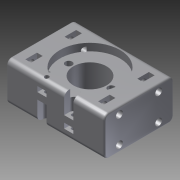
# Autodesk Inventor part: Z move middle
Saved by Autodesk Inventor 2012 (Build 160160000, 160)
## iProperties
Created: 2013-02-05
Part Number: Z move middle
Material: Default
Document SubType Name: Modeling
Designer: mce
Density: 1 g/cm^3
Mass: 44.0832 g
Surface Area: 145.334 cm^2
Volume: 44.0832 cm^3
Author: mce
Autodesk Inventor part; units mm, degrees
ref_plane "YZ Plane" through (0, 0, 0) normal (1, 0, 0) x (0, 1, 0)
ref_plane "XZ Plane" through (0, 0, 0) normal (0, 1, 0) x (-1, 0, 0)
ref_plane "XY Plane" through (0, 0, 0) normal (0, 0, 1) x (1, 0, 0)
sketch "Sketch1" plane through (0, 0, 0) normal (0, 0, 1) x (1, 0, 0)
  line L0 (0, 0) -> (60, 0)
  line L1 (60, 0) -> (60, 42.4)
  line L2 (60, 42.4) -> (0, 42.4)
  line L3 (0, 42.4) -> (0, 0)
  circle A0 centre (30, 21.2) radius 10.15
  dimension "d0" = 42.4
  dimension "d1" = 60
  dimension "d2" = 20.3
  dimension "d3" = 21.2
  dimension "d4" = 30
  constraints: 8 end point, 2 horizontal, 2 vertical, 1 centre point
  measures "d0" distance of L2.end L0.start
  measures "d1" distance of L0.start L0.end
  measures "d2" diameter of A0
  measures "d3" distance from line of L2 A0.centre
  measures "d4" distance from line of L3 A0.centre
extrude "Extrusion1" add sketch "Sketch1" along normal blind 24
sketch "Sketch2" plane through (0, 0, 0) normal (-1, 0, 0) x (0, 0, 1)
  line L0 (24, 0) -> (24, 42.4) projected
  line L1 (0, 42.4) -> (24, 42.4) projected
  line L2 (0, 42.4) -> (0, 0) projected
  line L3 (0, 0) -> (24, 0) projected
  circle A0 centre (4, 33.2) radius 2.1
  circle A1 centre (20, 33.2) radius 2.1
  circle A2 centre (20, 9.2) radius 2.1
  circle A3 centre (4, 9.2) radius 2.1
  dimension "d7" = 4.2
  dimension "d8" = 9.2
  dimension "d9" = 9.2
  dimension "d10" = 9.2
  dimension "d11" = 9.2
  dimension "d12" = 4
  dimension "d13" = 4
  dimension "d14" = 4
  dimension "d15" = 4
  constraints: 4 centre point, 3 equal radius
  measures "d7" diameter of A0
  measures "d8" distance from line of L1 A0.centre
  measures "d9" distance from line of L1 A1.centre
  measures "d10" distance from line of L3 A2.centre
  measures "d11" distance from line of L3 A3.centre
  measures "d12" distance from line of L2 A0.centre
  measures "d13" distance from line of L2 A3.centre
  measures "d14" distance from line of L0 A2.centre
  measures "d15" distance from line of L0 A1.centre
extrude "Extrusion2" cut sketch "Sketch2" against normal blind 16 contours A0 | A1 | A2 | A3
sketch "Sketch3" plane through (60, 0, 0) normal (1, 0, 0) x (0, 0, -1)
  line L0 (-24, 42.4) -> (-24, 0) projected
  line L1 (0, 0) -> (-24, 0) projected
  line L2 (0, 0) -> (0, 42.4) projected
  line L3 (0, 42.4) -> (-24, 42.4) projected
  circle A0 centre (-20, 33.2) radius 2.1
  circle A1 centre (-4, 33.2) radius 2.1
  circle A2 centre (-4, 9.2) radius 2.1
  circle A3 centre (-20, 9.2) radius 2.1
  dimension "d18" = 4.2
  dimension "d19" = 4
  dimension "d20" = 4
  dimension "d21" = 4
  dimension "d22" = 4
  dimension "d23" = 9.2
  dimension "d24" = 9.2
  dimension "d25" = 9.2
  dimension "d26" = 9.2
  constraints: 4 centre point, 3 equal radius
  measures "d18" diameter of A0
  measures "d19" distance from line of L0 A0.centre
  measures "d20" distance from line of L0 A3.centre
  measures "d21" distance from line of L2 A2.centre
  measures "d22" distance from line of L2 A1.centre
  measures "d23" distance from line of L3 A0.centre
  measures "d24" distance from line of L3 A1.centre
  measures "d25" distance from line of L1 A2.centre
  measures "d26" distance from line of L1 A3.centre
extrude "Extrusion3" cut sketch "Sketch3" against normal blind 16 contours A0 | A1 | A2 | A3
fillet "Fillet1" radius 3 4 edges at (30, 42.4, 0) (30, 0, 0) (30, 42.4, 24) (30, 0, 24)
fillet "Fillet2" radius 1 16 edges at (60, 21.2, 24) (60, 0.8787, 23.1213) (60, 0, 12) (60, 0.8787, 0.8787) (60, 21.2, 0) (60, 41.5213, 0.8787) (60, 42.4, 12) (60, 41.5213, 23.1213) (0, 41.5213, 23.1213) (0, 42.4, 12) (0, 41.5213, 0.8787) (0, 21.2, 0) (0, 0.8787, 0.8787) (0, 0, 12) (0, 0.8787, 23.1213) (0, 21.2, 24)
sketch "Sketch4" plane through (0, 0, 24) normal (0, 0, 1) x (1, 0, 0)
  line L0 (6, 36.75) -> (9.5, 36.75)
  line L1 (9.5, 36.75) -> (9.5, 29.65)
  line L2 (9.5, 29.65) -> (6, 29.65)
  line L3 (6, 29.65) -> (6, 36.75)
  line L4 (6, 12.75) -> (9.5, 12.75)
  line L5 (9.5, 12.75) -> (9.5, 5.65)
  line L6 (9.5, 5.65) -> (6, 5.65)
  line L7 (6, 5.65) -> (6, 12.75)
  line L8 (50.5, 36.75) -> (54, 36.75)
  line L9 (54, 36.75) -> (54, 29.65)
  line L10 (54, 29.65) -> (50.5, 29.65)
  line L11 (50.5, 29.65) -> (50.5, 36.75)
  line L12 (50.5, 12.75) -> (54, 12.75)
  line L13 (54, 12.75) -> (54, 5.65)
  line L14 (54, 5.65) -> (50.5, 5.65)
  line L15 (50.5, 5.65) -> (50.5, 12.75)
  line L16 (0, 39.4) -> (0, 3) projected
  line L17 (59, 42.4) -> (1, 42.4) projected
  line L18 (1, 0) -> (59, 0) projected
  line L19 (60, 3) -> (60, 39.4) projected
  point P0 (0, 0)
  dimension "d31" = 3.5
  dimension "d32" = 6
  dimension "d33" = 5.65
  dimension "d34" = 7.1
  dimension "d35" = 5.65
  dimension "d36" = 6
  constraints: 32 end point, 8 collinear, 4 equal length, 4 horizontal, 1 vertical
  measures "d31" distance of L0.start L0.end
  measures "d32" distance between parallel lines of L16 L3
  measures "d33" distance between parallel lines of L0 L17
  measures "d34" distance of L2.end L0.start
  measures "d35" distance between parallel lines of L6 L18
  measures "d36" distance between parallel lines of L9 L19
extrude "Extrusion4" cut sketch "Sketch4" against normal through all
sketch "Sketch5" plane through (0, 0, 24) normal (0, 0, 1) x (1, 0, 0)
  circle A0 centre (30, 21.2) radius 10.15 projected
  circle A1 centre (30, 21.2) radius 18.4
  point P0 (0, 0)
  dimension "d39" = 36.8
  constraints: 1 centre point, 1 coincident
  measures "d39" diameter of A1
extrude "Extrusion5" cut sketch "Sketch5" against normal blind 4.5
sketch "Sketch6" plane through (0, 0, 24) normal (0, 0, 1) x (1, 0, 0)
  circle A0 centre (17, 21.2) radius 2.1
  circle A1 centre (43, 21.2) radius 2.1
  line L0 (59, 42.4) -> (1, 42.4) projected
  line L1 (0, 39.4) -> (0, 3) projected
  point P0 (0, 0)
  dimension "d42" = 4.2
  dimension "d43" = 21.2
  dimension "d44" = 21.2
  dimension "d45" = 26
  dimension "d46" = 17
  constraints: 2 centre point, 1 equal radius
  measures "d42" diameter of A0
  measures "d43" distance from line of L0 A0.centre
  measures "d44" distance from line of L0 A1.centre
  measures "d45" distance of A1.centre A0.centre
  measures "d46" distance from line of L1 A0.centre
extrude "Extrusion6" cut sketch "Sketch6" against normal through all
sketch "Sketch7" plane through (0, 0, 0) normal (0, 0, -1) x (-1, 0, 0)
  circle A0 centre (-43, 21.2) radius 2.1 projected
  circle A1 centre (-17, 21.2) radius 2.1 projected
  line L0 (-43, 17.1008) -> (-46.55, 19.1504)
  line L1 (-46.55, 19.1504) -> (-46.55, 23.2496)
  line L2 (-46.55, 23.2496) -> (-43, 25.2992)
  line L3 (-43, 25.2992) -> (-39.45, 23.2496)
  line L4 (-39.45, 23.2496) -> (-39.45, 19.1504)
  line L5 (-39.45, 19.1504) -> (-43, 17.1008)
  line L6 (-13.45, 19.1504) -> (-17, 17.1008)
  line L7 (-17, 17.1008) -> (-20.55, 19.1504)
  line L8 (-20.55, 19.1504) -> (-20.55, 23.2496)
  line L9 (-20.55, 23.2496) -> (-17, 25.2992)
  line L10 (-17, 25.2992) -> (-13.45, 23.2496)
  line L11 (-13.45, 23.2496) -> (-13.45, 19.1504)
  point P0 (0, 0)
  point P1 (-46.55, 21.2)
  dimension "d49" = 7.1
  constraints: 24 end point, 2 coincident, 2 vertical, 1 equal length, 1 midpoint, 26 other
  measures "d49" distance between parallel lines of L1 L4
extrude "Extrusion7" cut sketch "Sketch7" against normal blind 5
sketch "Sketch8" plane through (0, 0, 5) normal (0, 0, -1) x (-1, 0, 0)
  circle A0 centre (-43, 21.2) radius 2.1 projected
  circle A1 centre (-43, 21.2) radius 2.1
  circle A2 centre (-17, 21.2) radius 2.1
  circle A3 centre (-17, 21.2) radius 2.1 projected
  point P0 (0, 0)
  constraints: 3 concentric, 2 centre point, 1 coincident
extrude "Extrusion8" add sketch "Sketch8" against normal blind 0.2
sketch "Sketch10" plane through (1, 0, 3) normal (0, -1, 0) x (1, 0, 0)
  line L0 (18, -3) -> (23.6, -3)
  line L1 (23.6, -3) -> (23.6, 9)
  line L2 (23.6, 9) -> (18, 9)
  line L3 (18, 9) -> (18, -3)
  line L4 (34.4, 21) -> (40, 21)
  line L5 (40, 21) -> (40, 9)
  line L6 (40, 9) -> (34.4, 9)
  line L7 (34.4, 9) -> (34.4, 21)
  line L8 (58, 21) -> (31.7055, 21) projected
  line L9 (0, -3) -> (58, -3) projected
  line L10 (-1, 18) -> (-1, 0) projected
  line L11 (59, 0) -> (59, 18) projected
  line L12 (18, 16.2) -> (23.6, 16.2)
  line L13 (23.6, 16.2) -> (23.6, 13)
  line L14 (23.6, 13) -> (18, 13)
  line L15 (18, 13) -> (18, 16.2)
  line L16 (34.4, 5) -> (40, 5)
  line L17 (40, 5) -> (40, 1.8)
  line L18 (40, 1.8) -> (34.4, 1.8)
  line L19 (34.4, 1.8) -> (34.4, 5)
  point P0 (-1, -3)
  dimension "d54" = 5.6
  dimension "d56" = 12
  dimension "d57" = 19
  dimension "d58" = 19
  dimension "d59" = 3.2
  dimension "d60" = 4
  dimension "d61" = 4
  constraints: 32 end point, 6 collinear, 4 vertical, 3 equal length, 3 horizontal
  measures "d54" distance of L1.end L2.end
  measures "d56" distance of L2.end L0.start
  measures "d57" distance between parallel lines of L10 L3
  measures "d58" distance between parallel lines of L11 L5
  measures "d59" distance between parallel lines of L12 L14
  measures "d60" distance between parallel lines of L14 L2
  measures "d61" distance between parallel lines of L16 L6
extrude "Extrusion9" cut sketch "Sketch10" against normal blind 6
sketch "Sketch11" plane through (0, 0, 24) normal (0, 0, 1) x (1, 0, 0)
  circle A0 centre (38.2, 3) radius 1.25
  circle A1 centre (21.8, 3) radius 1.25
  line L0 (1, 0) -> (35.4, 0) projected
  line L1 (41, 0) -> (35.4, 0) projected
  line L2 (35.4, 3) -> (35.4, 3.6102) projected
  line L3 (19, 0) -> (19, 6) projected
  point P0 (0, 0)
  point P1 (42.4, 6)
  dimension "d64" = 2.5
  dimension "d65" = 3
  dimension "d66" = 3
  dimension "d67" = 2.8
  dimension "d68" = 2.8
  constraints: 2 centre point, 1 equal radius, 1 other
  measures "d64" diameter of A0
  measures "d65" distance from line of A1.centre L0
  measures "d66" distance from line of L1 A0.centre
  measures "d68" distance from line of A1.centre L3
extrude "Extrusion10" cut sketch "Sketch11" against normal through all
fillet "Fillet3" radius 2.8 4 edges at (41, 6, 18) (35.4, 6, 15.75) (24.6, 6, 6) (19, 6, 6)
chamfer "Chamfer1" distance 1.5 angle 45 4 edges at (24.6, 6, 17.6) (19, 6, 17.6) (35.4, 6, 6.4) (41, 6, 6.4)
sketch "Sketch12" plane through (41, 0, 8) normal (0, 0, -1) x (-1, 0, 0)
  circle A0 centre (2.8, 3) radius 1.25 projected
  circle A1 centre (2.8, 3) radius 1.25
  point P0 (41, 0)
  constraints: 2 concentric, 1 centre point
extrude "Extrusion11" add sketch "Sketch12" against normal blind 0.2
sketch "Sketch13" plane through (24.6, 0, 12) normal (0, 0, -1) x (-1, 0, 0)
  circle A0 centre (2.8, 3) radius 1.25 projected
  circle A1 centre (2.8, 3) radius 1.25
  point P0 (24.6, 0)
  constraints: 2 concentric, 1 centre point
extrude "Extrusion12" add sketch "Sketch13" against normal blind 0.2
sketch "Sketch14" plane through (24.6, 0, 19.2) normal (0, 0, -1) x (-1, 0, 0)
  circle A0 centre (2.8, 3) radius 1.25 projected
  circle A1 centre (2.8, 3) radius 1.25
  point P0 (24.6, 0)
  constraints: 2 concentric, 1 centre point
extrude "Extrusion13" add sketch "Sketch14" against normal blind 0.2
equation "\"d57\" = d58"
body "Solid1"
